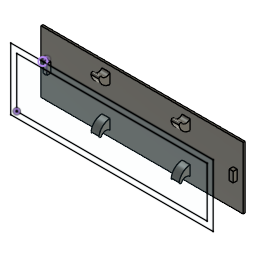
imu_box_v4 (Autodesk Fusion 360 design; units mm, degrees)
Autodesk Fusion 360 part; units mm, degrees
note: some values were not read from the file. Set by a fixed rule: which sketch regions a step uses.
sketch "Sketch1" plane through (0, 0, 0) normal (0, 1, 0) x (1, 0, 0)
  line L0 (0, 0) -> (95, 0)
  line L1 (95, 0) -> (95, -25)
  line L2 (95, -25) -> (0, -25)
  line L3 (0, -25) -> (0, 0)
  line L4 (98, 3) -> (98, -28)
  line L5 (98, -28) -> (-3, -28)
  line L6 (-3, -28) -> (-3, 3)
  line L7 (-3, 3) -> (98, 3)
  dimension "d1" = 95
  dimension "d2" = 25
  dimension "d3" = -3
  constraint horizontal L0
  constraint vertical L1
  constraint horizontal L2
  constraint vertical L3
  constraint coincident L0.start L3.end
  measures "d1" distance of L1.end L2.end
  measures "d2" distance of L0.end L1.end
extrude "Extrude1" add sketch "Sketch1" along normal blind 15 makes body 1
extrude "Extrude2" add sketch "Sketch1" along normal blind 3 contours L0 L1 L2 L3 bodies 1
ref_plane "WorkPlane1" through (47.5, 7.5, 12.5) normal (0, 0, 1) x (1, 0, 0)
ref_plane "WorkPlane2" through (47.5, 7.5, 12.5) normal (1, 0, 0) x (0, 0, -1)
sketch "Sketch3" plane through (47.5, 0, 0) normal (1, 0, 0) x (0, 1, 0)
  line L0 (15, 28) -> (0, 28)
  line L1 (0, 28) -> (0, -3)
  line L2 (0, -3) -> (15, -3)
  line L3 (15, -3) -> (15, 0)
  line L4 (15, 0) -> (3, 0)
  line L5 (3, 0) -> (3, 25)
  line L6 (3, 25) -> (15, 25)
  line L7 (15, 25) -> (15, 28)
  circle A0 centre (10.2546, 25) radius 0.75
  circle A1 centre (10.2546, 25) radius 0.85
  arc A2 (9.5155, 24.8723) -> (15, 19.8539) centre (15.4085, 25.8065) ccw
  arc A3 (11.0046, 25) -> (15, 25) centre (13.0023, 26.5886) ccw
  line L8 (20.7, 12.5) -> (-5.7, 12.5)
  line L9 (15, 28) -> (15, -3)
  line L10 (15, 28) -> (16, 28)
  line L11 (16, 28) -> (16, -3)
  line L12 (15, -3) -> (16, -3)
  arc A4 (15, 0) -> (11.0046, 0) centre (13.0023, -1.5886) ccw
  arc A5 (15, 5.1461) -> (9.5155, 0.1277) centre (15.4085, -0.8065) ccw
  circle A6 centre (10.2546, 0) radius 0.75
  circle A7 centre (10.2546, 0) radius 0.85
  dimension "d8" = 1.5
  constraint coincident L6 A0.centre
  constraint coincident A0 A2.start
  constraint coincident A0 A3.start
  constraint concentric A0 A1
  constraint coincident L6.end L7.start
  constraint coincident L6 A3.start
  constraint coincident L0.start L7.end
  constraint coincident L2.end L3.start
  constraint coincident A2.end L9
  constraint perpendicular L7 L10
  constraint perpendicular L10 L11
  constraint symmetric A0 L8 A6
  constraint symmetric A1 L8 A7
  constraint symmetric A2.end L8 A5.start
  constraint symmetric A2 L8 A5
  constraint symmetric A3 L8 A4
  constraint symmetric A3.start L8 A4.end
  constraint symmetric A2.start L8 A5.end
  constraint symmetric L8 L6.end L3.end
  measures "d8" diameter of A0
extrude "Extrude9" cut sketch "Sketch3" along normal mid plane 95 contours L6 A1 A3 | L6 A0 A1 | A0 A1 A2 A3 | L6 A0 | L6 A0 | L6 A0 A1 A2 | L4 A5 A6 A7 | L4 A6 A7 | A4 A5 A6 A7 | L4 A4 A7 | L4 A6 | L4 A6 picked at (11.048, 24.9876) picked at (11.048, 0.0124) bodies 1
extrude "Extrude10" add sketch "Sketch3" along normal blind 4 from surface at 20 separate body contours A1 A2 A3 L9 | A0 A1 A2 A3 | L6 A0 | L6 A0 | L9 A4 A5 A7 | A4 A5 A6 A7 | L4 A6 | L4 A6 makes body 2 at (68.8333, 9.9277, 23.4484) makes body 3 at (68.8333, 11.2723, 3.4937)
extrude "Extrude11" add sketch "Sketch3" along normal blind 4 from surface at -20 separate body contours A1 A2 A3 L9 | A0 A1 A2 A3 | L6 A0 | L6 A0 | L9 A4 A5 A7 | A4 A5 A6 A7 | L4 A6 | L4 A6 makes body 4 at (28.8333, 11.2723, 3.4937) makes body 5 at (28.8333, 9.9277, 23.4484)
extrude "Extrude12" add sketch "Sketch3" along normal mid plane 101 separate body contours L7 L8 L9 L10 L11 | L3 L8 L9 L11 L12 makes body 6
sketch "Sketch6" plane through (0, 15, 0) normal (0, 1, 0) x (1, 0, 0)
  line L0 (-3, -25) -> (-3, -28)
  line L1 (98, -28) -> (98, -25)
  line L2 (95, -25) -> (0, -25)
  line L3 (0, -25) -> (0, 0)
  line L4 (0, 0) -> (95, 0)
  line L5 (95, -25) -> (95, 0)
  line L6 (0, -14.9882) -> (2, -14.9882)
  line L7 (2, -14.9882) -> (2, -9.9882)
  line L8 (2, -9.9882) -> (0, -9.9882)
  line L9 (0, -14.9882) -> (0, -9.9882)
  line L10 (0, -14.9882) -> (0, -9.9882)
  line L11 (95, -9.9882) -> (93, -9.9882)
  line L12 (93, -9.9882) -> (93, -14.9882)
  line L13 (93, -14.9882) -> (95, -14.9882)
  line L14 (95, -9.9882) -> (95, -14.9882)
  line L15 (98, -25) -> (71.5, -25)
  line L16 (-3, -28) -> (98, -28)
  line L17 (71.5, -25) -> (67.5, -25)
  line L18 (67.5, -25) -> (31.5, -25)
  line L19 (31.5, -25) -> (27.5, -25)
  line L20 (27.5, -25) -> (-3, -25)
  constraint coincident L3 L6.start
  constraint perpendicular L3 L6
  constraint perpendicular L6 L7
  constraint coincident L3 L8.end
  constraint perpendicular L3 L8
  constraint coincident L5 L11.start
  constraint perpendicular L5 L11
  constraint perpendicular L11 L12
  constraint coincident L5 L13.end
  constraint perpendicular L5 L13
extrude "Extrude8" add sketch "Sketch6" against normal blind 2 contours L3 L6 L7 L8 L9 L10 | L5 L11 L12 L13 L14 bodies 6
sketch "Sketch7" plane through (0, 0, 0) normal (-1, 0, 0) x (0, -1, 0)
  line L0 (-13, 14.9882) -> (-15, 14.9882)
  line L1 (-13, 9.9882) -> (-13, 14.9882)
  line L2 (-15, 9.9882) -> (-13, 9.9882)
  line L3 (-15, 14.9882) -> (-15, 9.9882)
move_face "OffsetFaces1" offset -0.2 1 faces at (0, 14.3333, 13.3216) on bodies 6
hidden bodies 1
